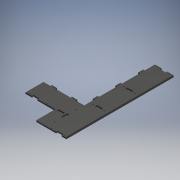
# Autodesk Inventor part: BA10
Saved by Autodesk Inventor 2017 (Build 210142000, 142)
## iProperties
Created: 2019-05-29
Part Number: BA10
Material: Wood (Cherry)
Document SubType Name: Modeling
Designer: Dell
Density: 0.63 g/cm^3
Appearance: Smooth - Black
Mass: 296.487 g
Surface Area: 1614.58 cm^2
Volume: 470.615 cm^3
Author: Dell
Autodesk Inventor part; units mm, degrees
ref_plane "YZ Plane" through (0, 0, 0) normal (1, 0, 0) x (0, 1, 0)
ref_plane "XZ Plane" through (0, 0, 0) normal (0, 1, 0) x (-1, 0, 0)
ref_plane "XY Plane" through (0, 0, 0) normal (0, 0, 1) x (1, 0, 0)
sketch "Sketch1" plane through (0, 0, 0) normal (0, 0, 1) x (1, 0, 0)
  line L0 (0, 0) -> (0, 355.6)
  line L1 (0, 355.6) -> (95.25, 355.6)
  line L2 (95.25, 355.6) -> (95.25, -184.15)
  line L3 (95.25, -184.15) -> (-208.3092, -184.15) construction
  line L4 (-208.3092, -184.15) -> (-208.3092, 0) construction
  line L5 (-208.3092, 0) -> (0, 0)
  line L6 (-208.3092, -184.15) -> (-55.9092, -184.15) construction
  line L7 (-55.9092, -184.15) -> (-55.9092, -88.9)
  line L8 (-55.9092, -88.9) -> (-208.3092, -88.9)
  line L9 (-208.3092, -88.9) -> (-208.3092, -184.15) construction
  line L10 (-208.3092, -88.9) -> (-208.3092, 0)
  line L11 (-55.9092, -184.15) -> (95.25, -184.15)
  line L12 (0, 304.8) -> (-7.62, 304.8)
  line L13 (-7.62, 304.8) -> (-7.62, 279.4)
  line L14 (-7.62, 279.4) -> (0, 279.4)
  line L15 (0, 279.4) -> (0, 304.8)
  line L16 (0, 165.1) -> (-7.62, 165.1)
  line L17 (-7.62, 165.1) -> (-7.62, 190.5)
  line L18 (-7.62, 190.5) -> (0, 190.5)
  line L19 (0, 190.5) -> (0, 165.1)
  line L20 (0, 76.2) -> (-7.62, 76.2)
  line L21 (-7.62, 76.2) -> (-7.62, 50.8)
  line L22 (-7.62, 50.8) -> (0, 50.8)
  line L23 (0, 50.8) -> (0, 76.2)
  line L24 (-6.35, -79.375) -> (0, -79.375)
  line L25 (0, -79.375) -> (0, -104.775)
  line L26 (0, -104.775) -> (-6.35, -104.775)
  line L27 (-6.35, -104.775) -> (-6.35, -79.375)
  line L28 (-7.62, -78.105) -> (1.27, -78.105)
  line L29 (1.27, -78.105) -> (1.27, -106.045)
  line L30 (1.27, -106.045) -> (-7.62, -106.045)
  line L31 (-7.62, -106.045) -> (-7.62, -78.105)
  point P0 (0, 177.8)
  point P1 (0, -92.075)
  point P2 (-6.35, -92.075)
  point P3 (-7.62, -92.075)
  point P4 (-3.175, -79.375)
  point P5 (-3.175, -78.105)
  point P6 (-208.3092, -92.075)
  dimension "d0" = 95.25
  dimension "d1" = 355.6
  dimension "d2" = 303.5592
  dimension "d3" = 184.15
  dimension "d4" = 152.4
  dimension "d5" = 95.25
  dimension "d6" = 7.62
  dimension "d7" = 25.4
  dimension "d8" = 25.4
  dimension "d9" = 25.4
  dimension "d10" = 50.8
  dimension "d11" = 50.8
  dimension "d12" = 6.35
  dimension "d13" = 25.4
  dimension "d14" = 1.27
  dimension "d15" = 1.27
  constraints: 64 end point, 12 parallel, 10 perpendicular, 8 midpoint, 7 horizontal, 4 point on line, 3 vertical alignment, 2 horizontal alignment, 2 vertical, 1 collinear
  measures "d0" distance between parallel lines of L2 L0
  measures "d1" distance of L0.start L0.end
  measures "d2" distance between parallel lines of L4 L2
  measures "d3" distance of L3.end L4.end
  measures "d4" distance of L7.end L8.end
  measures "d5" distance of L6.end L7.end
  measures "d6" distance of L14.end L13.end
  measures "d7" distance of L12.end L13.end
  measures "d8" distance of L16.end L17.end
  measures "d9" distance of L20.end L21.end
  measures "d10" distance between parallel lines of L1 L12
  measures "d11" distance between parallel lines of L5 L22
  measures "d12" distance of L25.end L26.end
  measures "d13" distance of L24.end L25.end
  measures "d14" distance between parallel lines of L28 L24
  measures "d15" distance between parallel lines of L29 L25
extrude "Extrusion1" add sketch "Sketch1" along normal blind 6.35 contours L0 L1 L2 L11 L7 L8 L10 L5 | L22 L21 L20 L0 | L16 L17 L18 L0 | L14 L13 L12 L0
sketch "Sketch3" plane through (0, 355.6, 0) normal (0, 1, 0) x (1, 0, 0)
  line L0 (95.25, 0) -> (95.25, -6.35) projected
  line L1 (95.25, 0) -> (91.5838, -6.35)
  line L2 (91.5838, -6.35) -> (95.25, -6.35)
  line L3 (95.25, -6.35) -> (91.5838, -6.35)
  line L4 (-208.3092, 0) -> (-208.3092, -6.35)
  line L5 (-208.3092, -6.35) -> (-204.6431, -6.35)
  line L6 (-208.3092, 0) -> (-208.3092, -6.35) projected
  line L7 (-204.6431, -6.35) -> (-208.3092, 0)
  line L8 (0, -6.35) -> (-208.3092, -6.35) projected
  line L9 (95.25, -6.35) -> (0, -6.35) projected
  dimension "d23" = 30
  dimension "d24" = 30
  constraints: 12 end point, 2 point on line, 1 collinear, 1 vertical
  measures "d23" angle of L0 L1
  measures "d24" angle of L4 L7
extrude "Extrusion2" cut sketch "Sketch3" against normal through all
sketch "Sketch4" plane through (0, 0, 6.35) normal (0, 0, 1) x (1, 0, 0)
  line L0 (-55.9092, -184.15) -> (91.5838, -184.15) projected
  line L1 (44.45, -184.15) -> (69.85, -184.15)
  line L2 (69.85, -184.15) -> (69.85, -176.53)
  line L3 (69.85, -176.53) -> (44.45, -176.53)
  line L4 (44.45, -176.53) -> (44.45, -184.15)
  line L5 (-7.62, -106.045) -> (-7.62, -78.105) projected
  point P0 (0, 0)
  dimension "d25" = 25.4
  dimension "d26" = 7.62
  dimension "d27" = 52.07
  constraints: 8 end point, 2 parallel, 1 horizontal, 1 perpendicular, 1 point on line
  measures "d25" distance of L3.end L2.end
  measures "d26" distance of L2.end L1.end
  measures "d27" distance between parallel lines of L4 L5
extrude "Extrusion3" cut sketch "Sketch4" against normal through all
sketch "Sketch5" plane through (0, 0, 6.35) normal (0, 0, 1) x (1, 0, 0)
  line L0 (33.0919, 355.6) -> (58.4919, 355.6)
  line L1 (58.4919, 355.6) -> (58.4919, 347.98)
  line L2 (58.4919, 347.98) -> (33.0919, 347.98)
  line L3 (33.0919, 347.98) -> (33.0919, 355.6)
  line L4 (91.5838, 355.6) -> (0, 355.6) projected
  point P0 (0, 0)
  point P1 (45.7919, 355.6)
  dimension "d30" = 7.62
  dimension "d31" = 25.4
  constraints: 8 end point, 2 midpoint, 2 parallel, 1 horizontal, 1 perpendicular
  measures "d30" distance of L2.end L0.start
  measures "d31" distance of L1.end L2.end
extrude "Extrusion4" cut sketch "Sketch5" against normal through all
sketch "Sketch6" plane through (0, 0, 6.35) normal (0, 0, 1) x (1, 0, 0)
  line L0 (33.0919, 31.75) -> (58.4919, 31.75)
  line L1 (58.4919, 31.75) -> (58.4919, 25.4)
  line L2 (58.4919, 25.4) -> (33.0919, 25.4)
  line L3 (33.0919, 25.4) -> (33.0919, 31.75)
  line L4 (-55.9092, -184.15) -> (44.45, -184.15) projected
  line L5 (58.4919, 347.98) -> (33.0919, 347.98) projected
  point P0 (0, 0)
  point P1 (45.7919, 31.75)
  point P2 (45.7919, 347.98)
  dimension "d34" = 25.4
  dimension "d35" = 6.35
  dimension "d36" = 209.55
  constraints: 8 end point, 2 midpoint, 2 parallel, 1 horizontal, 1 perpendicular, 1 vertical alignment
  measures "d34" distance of L1.end L2.end
  measures "d35" distance of L0.end L1.end
  measures "d36" distance between parallel lines of L4 L2
extrude "Extrusion5" cut sketch "Sketch6" against normal through all
sketch "Sketch7" plane through (0, 0, 6.35) normal (0, 0, 1) x (1, 0, 0)
  line L0 (33.0919, 184.15) -> (58.4919, 184.15)
  line L1 (58.4919, 184.15) -> (58.4919, 177.8)
  line L2 (58.4919, 177.8) -> (33.0919, 177.8)
  line L3 (33.0919, 177.8) -> (33.0919, 184.15)
  line L4 (58.4919, 347.98) -> (33.0919, 347.98) projected
  line L5 (33.0919, 355.6) -> (0, 355.6) projected
  point P0 (0, 0)
  point P1 (45.7919, 184.15)
  point P2 (45.7919, 347.98)
  dimension "d39" = 25.4
  dimension "d40" = 6.35
  dimension "d41" = 177.8
  constraints: 8 end point, 2 midpoint, 2 parallel, 1 horizontal, 1 perpendicular, 1 vertical alignment
  measures "d39" distance of L1.end L2.end
  measures "d40" distance of L0.end L1.end
  measures "d41" distance between parallel lines of L5 L2
extrude "Extrusion6" cut sketch "Sketch7" against normal through all
sketch "Sketch8" plane through (0, 0, 6.35) normal (0, 0, 1) x (1, 0, 0)
  line L0 (-170.2092, 0) -> (-144.8092, 0)
  line L1 (-144.8092, 0) -> (-144.8092, 7.62)
  line L2 (-144.8092, 7.62) -> (-170.2092, 7.62)
  line L3 (-170.2092, 7.62) -> (-170.2092, 0)
  line L4 (-68.6092, 0) -> (-43.2092, 0)
  line L5 (-43.2092, 0) -> (-43.2092, 7.62)
  line L6 (-43.2092, 7.62) -> (-68.6092, 7.62)
  line L7 (-68.6092, 7.62) -> (-68.6092, 0)
  line L8 (-157.5092, 7.62) -> (-55.9092, 7.62) construction
  line L9 (0, 0) -> (-208.3092, 0) projected
  dimension "d44" = 25.4
  dimension "d45" = 7.62
  dimension "d46" = 25.4
  dimension "d47" = 7.62
  dimension "d48" = 101.6
  dimension "d51" = 38.1
  constraints: 18 end point, 4 parallel, 2 horizontal, 2 midpoint, 2 perpendicular, 2 point on line
  measures "d44" distance of L2.end L1.end
  measures "d45" distance of L1.end L0.end
  measures "d46" distance of L6.end L5.end
  measures "d47" distance of L5.end L4.end
  measures "d48" distance of L8.start L8.end
  measures "d51" horizontal distance of L2.end L9.end
extrude "Extrusion7" add sketch "Sketch8" against normal blind 6.35
sketch "Sketch9" plane through (0, 0, 6.35) normal (0, 0, 1) x (1, 0, 0)
  line L0 (33.0919, 28.575) -> (0, 28.575) construction
  line L1 (0, 50.8) -> (0, 0) construction
  line L2 (58.4919, 28.575) -> (91.5838, 28.575) construction
  line L3 (91.5838, -184.15) -> (91.5838, 355.6) construction
  circle A0 centre (16.546, 28.575) radius 2.25
  circle A1 centre (75.0379, 28.575) radius 2.25
  line L4 (33.0919, 25.4) -> (33.0919, 31.75) projected
  line L5 (58.4919, 31.75) -> (58.4919, 25.4) projected
  circle A2 centre (16.546, 180.975) radius 2.25
  circle A3 centre (75.0379, 180.975) radius 2.25
  line L6 (58.4919, 184.15) -> (58.4919, 177.8) projected
  circle A4 centre (16.546, 351.79) radius 2.25
  circle A5 centre (75.0379, 351.79) radius 2.25
  line L7 (33.0919, 347.98) -> (33.0919, 355.6) projected
  circle A6 centre (-3.175, -39.0525) radius 2.25
  circle A7 centre (-3.175, -145.0975) radius 2.25
  line L8 (1.27, -106.045) -> (-7.62, -106.045) construction
  line L9 (-7.62, -78.105) -> (1.27, -78.105) construction
  line L10 (-3.175, -78.105) -> (-3.175, 0) construction
  line L11 (-3.175, -106.045) -> (-3.175, -184.15) construction
  line L12 (-55.9092, -184.15) -> (44.45, -184.15) construction
  line L13 (0, 0) -> (-43.2092, 0) projected
  circle A8 centre (-157.5092, 3.81) radius 2.25
  circle A9 centre (-55.9092, 3.81) radius 2.25
  circle A10 centre (-3.81, 63.5) radius 2.25
  circle A11 centre (-3.81, 177.8) radius 2.25
  circle A12 centre (-3.81, 292.1) radius 2.25
  line L14 (-144.8092, 7.62) -> (-170.2092, 7.62) projected
  line L15 (-43.2092, 7.62) -> (-68.6092, 7.62) projected
  line L16 (-7.62, 304.8) -> (-7.62, 279.4) projected
  line L17 (-7.62, 190.5) -> (-7.62, 165.1) projected
  line L18 (-7.62, 76.2) -> (-7.62, 50.8) projected
  line L19 (-68.6092, 7.62) -> (-68.6092, 0) projected
  line L20 (-7.62, 50.8) -> (0, 50.8) projected
  circle A13 centre (16.546, -180.34) radius 2.25
  circle A14 centre (80.7169, -180.34) radius 2.25
  line L21 (69.85, -176.53) -> (69.85, -184.15) projected
  line L22 (69.85, -180.34) -> (91.5838, -180.34) construction
  point P0 (58.4919, 180.975)
  point P1 (33.0919, 351.79)
  point P2 (-3.175, -145.0975)
  point P3 (-157.5092, 7.62)
  point P4 (-55.9092, 7.62)
  point P5 (-7.62, 292.1)
  point P6 (-7.62, 177.8)
  point P7 (-7.62, 63.5)
  point P8 (-68.6092, 3.81)
  point P9 (-3.81, 50.8)
  dimension "d52" = 4.5
  dimension "d53" = 4.5
  dimension "d54" = 4.5
  dimension "d55" = 4.5
  dimension "d56" = 4.5
  dimension "d57" = 4.5
  dimension "d58" = 4.5
  dimension "d59" = 4.5
  dimension "d60" = 4.5
  dimension "d61" = 4.5
  dimension "d62" = 4.5
  dimension "d63" = 4.5
  dimension "d64" = 4.5
  dimension "d65" = 4.5
  dimension "d66" = 4.5
  constraints: 19 midpoint, 15 centre point, 12 vertical alignment, 11 horizontal alignment, 10 end point, 7 point on line, 3 coincident, 2 vertical, 1 horizontal, 1 perpendicular
  measures "d52" diameter of A0
  measures "d53" diameter of A1
  measures "d54" diameter of A2
  measures "d55" diameter of A3
  measures "d56" diameter of A4
  measures "d57" diameter of A5
  measures "d58" diameter of A6
  measures "d59" diameter of A7
  measures "d60" diameter of A8
  measures "d61" diameter of A9
  measures "d62" diameter of A10
  measures "d63" diameter of A11
  measures "d64" diameter of A12
  measures "d65" diameter of A13
  measures "d66" diameter of A14
extrude "Extrusion8" cut sketch "Sketch9" against normal through all
sketch "Sketch10" plane through (0, 0, 6.35) normal (0, 0, 1) x (1, 0, 0)
  line L0 (-171.4646, -82.55) -> (-146.0646, -82.55)
  line L1 (-146.0646, -82.55) -> (-146.0646, -88.9)
  line L2 (-146.0646, -88.9) -> (-171.4646, -88.9)
  line L3 (-171.4646, -88.9) -> (-171.4646, -82.55)
  line L4 (-19.0646, -82.55) -> (-44.4646, -82.55)
  line L5 (-44.4646, -82.55) -> (-44.4646, -88.9)
  line L6 (-44.4646, -88.9) -> (-19.0646, -88.9)
  line L7 (-19.0646, -88.9) -> (-19.0646, -82.55)
  line L8 (-55.9092, -184.15) -> (44.45, -184.15) projected
  line L9 (-204.6431, -88.9) -> (-55.9092, -88.9) projected
  line L10 (58.4919, 25.4) -> (33.0919, 25.4) projected
  line L11 (-55.9092, -88.9) -> (-7.62, -88.9) construction
  line L12 (-7.62, -78.105) -> (-7.62, -106.045) projected
  point P0 (0, 0)
  point P1 (45.7919, 25.4)
  point P2 (-31.7646, -88.9)
  dimension "d70" = 6.35
  dimension "d71" = 25.4
  dimension "d72" = 25.4
  dimension "d73" = 101.6
  constraints: 18 end point, 4 parallel, 4 point on line, 3 horizontal, 3 midpoint, 2 perpendicular
  measures "d70" distance of L2.end L0.start
  measures "d71" distance of L0.start L0.end
  measures "d72" distance of L4.start L4.end
  measures "d73" distance of L4.end L0.end
extrude "Extrusion9" cut sketch "Sketch10" against normal through all
sketch "Sketch11" plane through (0, 0, 6.35) normal (0, 0, 1) x (1, 0, 0)
  circle A0 centre (-100.9869, -85.725) radius 2.25
  circle A1 centre (-188.0538, -85.725) radius 2.25
  line L0 (-204.6431, -88.9) -> (-171.4646, -88.9) projected
  line L1 (-146.0646, -88.9) -> (-55.9092, -88.9) projected
  line L2 (-171.4646, -88.9) -> (-171.4646, -82.55) projected
  point P0 (0, 0)
  point P1 (-188.0538, -88.9)
  point P2 (-100.9869, -88.9)
  point P3 (-171.4646, -85.725)
  point P4 (-171.4646, -85.725)
  dimension "d76" = 4.5
  dimension "d77" = 4.5
  constraints: 4 midpoint, 2 centre point, 2 horizontal alignment, 2 vertical alignment
  measures "d76" diameter of A0
  measures "d77" diameter of A1
extrude "Extrusion10" cut sketch "Sketch11" against normal through all
sketch "Sketch12" plane through (0, 0, 6.35) normal (0, 0, 1) x (1, 0, 0)
  line L0 (33.0919, 355.6) -> (0, 355.6) projected
  line L1 (31.8219, 355.6) -> (59.7619, 355.6)
  line L2 (59.7619, 355.6) -> (59.7619, 347.98)
  line L3 (59.7619, 347.98) -> (31.8219, 347.98)
  line L4 (31.8219, 347.98) -> (31.8219, 355.6)
  line L5 (31.8219, 185.42) -> (59.7619, 185.42)
  line L6 (59.7619, 185.42) -> (59.7619, 176.53)
  line L7 (59.7619, 176.53) -> (31.8219, 176.53)
  line L8 (31.8219, 176.53) -> (31.8219, 185.42)
  line L9 (31.8219, 33.02) -> (59.7619, 33.02)
  line L10 (59.7619, 33.02) -> (59.7619, 24.13)
  line L11 (59.7619, 24.13) -> (31.8219, 24.13)
  line L12 (31.8219, 24.13) -> (31.8219, 33.02)
  line L13 (-204.6431, -88.9) -> (-171.4646, -88.9) projected
  line L14 (-172.7346, -88.9) -> (-144.7946, -88.9)
  line L15 (-144.7946, -88.9) -> (-144.7946, -81.28)
  line L16 (-144.7946, -81.28) -> (-172.7346, -81.28)
  line L17 (-172.7346, -81.28) -> (-172.7346, -88.9)
  line L18 (-45.7346, -81.28) -> (-17.7946, -81.28)
  line L19 (-17.7946, -81.28) -> (-17.7946, -90.17)
  line L20 (-17.7946, -90.17) -> (-45.7346, -90.17)
  line L21 (-45.7346, -90.17) -> (-45.7346, -81.28)
  line L22 (-55.9092, -184.15) -> (44.45, -184.15) projected
  line L23 (43.18, -184.15) -> (71.12, -184.15)
  line L24 (71.12, -184.15) -> (71.12, -176.53)
  line L25 (71.12, -176.53) -> (43.18, -176.53)
  line L26 (43.18, -176.53) -> (43.18, -184.15)
  line L27 (-171.4646, -82.55) -> (-146.0646, -82.55) projected
  line L28 (-171.4646, -88.9) -> (-171.4646, -82.55) projected
  line L29 (-44.4646, -88.9) -> (-44.4646, -82.55) projected
  line L30 (33.0919, 25.4) -> (33.0919, 31.75) projected
  line L31 (58.4919, 31.75) -> (33.0919, 31.75) projected
  line L32 (33.0919, 177.8) -> (33.0919, 184.15) projected
  line L33 (33.0919, 184.15) -> (58.4919, 184.15) projected
  line L34 (58.4919, 347.98) -> (33.0919, 347.98) projected
  line L35 (44.45, -176.53) -> (69.85, -176.53) projected
  line L36 (44.45, -184.15) -> (44.45, -176.53) projected
  line L37 (-19.0646, -88.9) -> (-44.4646, -88.9) projected
  point P0 (0, 0)
  point P1 (-158.7646, -82.55)
  point P2 (-158.7646, -82.55)
  point P3 (-158.7646, -81.28)
  point P4 (45.7919, 347.98)
  point P5 (45.7919, 184.15)
  point P6 (45.7919, 185.42)
  point P7 (33.0919, 180.975)
  point P8 (31.8219, 180.975)
  point P9 (33.0919, 28.575)
  point P10 (31.8219, 28.575)
  point P11 (45.7919, 31.75)
  point P12 (45.7919, 33.02)
  point P13 (57.15, -176.53)
  point P14 (-31.7646, -88.9)
  point P15 (-31.7646, -90.17)
  point P16 (-44.4646, -85.725)
  point P17 (-45.7346, -85.725)
  dimension "d80" = 1.27
  dimension "d81" = 1.27
  dimension "d82" = 1.27
  dimension "d83" = 1.27
  dimension "d84" = 1.27
  dimension "d85" = 1.27
  dimension "d86" = 1.27
  dimension "d87" = 1.27
  constraints: 48 end point, 19 midpoint, 12 parallel, 6 horizontal, 6 perpendicular, 6 point on line, 4 vertical alignment, 3 horizontal alignment
  measures "d80" distance from line of L27 L15.end
  measures "d81" distance between parallel lines of L17 L28
  measures "d82" distance between parallel lines of L21 L29
  measures "d83" distance between parallel lines of L12 L30
  measures "d84" distance from line of L9.end L31
  measures "d85" distance between parallel lines of L8 L32
  measures "d86" distance between parallel lines of L33 L5
  measures "d87" distance between parallel lines of L26 L36
extrude "Extrusion11" cut sketch "Sketch12" against normal through all
sketch "Sketch13" plane through (0, 0, 6.35) normal (0, 0, 1) x (1, 0, 0)
  line L0 (71.12, -176.53) -> (71.12, -184.15) construction
  line L1 (71.12, -184.15) -> (91.5838, -184.15) construction
  line L2 (91.5838, -184.15) -> (91.5838, 355.6) construction
  line L3 (91.5838, 355.6) -> (59.7619, 355.6) construction
  line L4 (59.7619, 355.6) -> (59.7619, 347.98) construction
  line L5 (59.7619, 347.98) -> (31.8219, 347.98) construction
  line L6 (31.8219, 347.98) -> (31.8219, 355.6) construction
  line L7 (31.8219, 355.6) -> (0, 355.6) construction
  line L8 (0, 355.6) -> (0, 304.8) construction
  line L9 (0, 304.8) -> (-7.62, 304.8) construction
  line L10 (-7.62, 304.8) -> (-7.62, 279.4) construction
  line L11 (-7.62, 279.4) -> (0, 279.4) construction
  line L12 (0, 279.4) -> (0, 190.5) construction
  line L13 (0, 190.5) -> (-7.62, 190.5) construction
  line L14 (-7.62, 190.5) -> (-7.62, 165.1) construction
  line L15 (-7.62, 165.1) -> (0, 165.1) construction
  line L16 (0, 165.1) -> (0, 76.2) construction
  line L17 (0, 76.2) -> (-7.62, 76.2) construction
  line L18 (-7.62, 76.2) -> (-7.62, 50.8) construction
  line L19 (-7.62, 50.8) -> (0, 50.8) construction
  line L20 (0, 50.8) -> (0, 0) construction
  line L21 (0, 0) -> (-43.2092, 0) construction
  line L22 (-43.2092, 0) -> (-43.2092, 7.62) construction
  line L23 (-43.2092, 7.62) -> (-68.6092, 7.62) construction
  line L24 (-68.6092, 7.62) -> (-68.6092, 0) construction
  line L25 (-68.6092, 0) -> (-144.8092, 0) construction
  line L26 (-144.8092, 0) -> (-144.8092, 7.62) construction
  line L27 (-144.8092, 7.62) -> (-170.2092, 7.62) construction
  line L28 (-170.2092, 7.62) -> (-170.2092, 0) construction
  line L29 (-170.2092, 0) -> (-204.6431, 0) construction
  line L30 (-204.6431, 0) -> (-204.6431, -88.9) construction
  line L31 (-204.6431, -88.9) -> (-172.7346, -88.9) construction
  line L32 (-172.7346, -88.9) -> (-172.7346, -81.28) construction
  line L33 (-172.7346, -81.28) -> (-144.7946, -81.28) construction
  line L34 (-144.7946, -81.28) -> (-144.7946, -88.9) construction
  line L35 (-144.7946, -88.9) -> (-55.9092, -88.9) construction
  line L36 (-55.9092, -88.9) -> (-55.9092, -184.15) construction
  line L37 (-55.9092, -184.15) -> (43.18, -184.15) construction
  line L38 (43.18, -184.15) -> (43.18, -176.53) construction
  line L39 (43.18, -176.53) -> (71.12, -176.53) construction
  line L40 (31.8219, 24.13) -> (31.8219, 33.02) construction
  line L41 (31.8219, 33.02) -> (59.7619, 33.02) construction
  line L42 (59.7619, 33.02) -> (59.7619, 24.13) construction
  line L43 (59.7619, 24.13) -> (31.8219, 24.13) construction
  line L44 (31.8219, 176.53) -> (31.8219, 185.42) construction
  line L45 (31.8219, 185.42) -> (59.7619, 185.42) construction
  line L46 (59.7619, 185.42) -> (59.7619, 176.53) construction
  line L47 (59.7619, 176.53) -> (31.8219, 176.53) construction
  line L48 (-45.7346, -90.17) -> (-45.7346, -81.28) construction
  line L49 (-45.7346, -81.28) -> (-17.7946, -81.28) construction
  line L50 (-17.7946, -81.28) -> (-17.7946, -90.17) construction
  line L51 (-17.7946, -90.17) -> (-45.7346, -90.17) construction
  circle A0 centre (-100.9869, -85.725) radius 2.25 construction
  circle A1 centre (-188.0538, -85.725) radius 2.25 construction
  circle A2 centre (16.546, -180.34) radius 2.25 construction
  circle A3 centre (-3.81, 177.8) radius 2.25 construction
  circle A4 centre (-55.9092, 3.81) radius 2.25 construction
  circle A5 centre (-3.175, -145.0975) radius 2.25 construction
  circle A6 centre (75.0379, 351.79) radius 2.25 construction
  circle A7 centre (75.0379, 180.975) radius 2.25 construction
  circle A8 centre (75.0379, 28.575) radius 2.25 construction
  circle A9 centre (16.546, 28.575) radius 2.25 construction
  circle A10 centre (16.546, 180.975) radius 2.25 construction
  circle A11 centre (16.546, 351.79) radius 2.25 construction
  circle A12 centre (-3.175, -39.0525) radius 2.25 construction
  circle A13 centre (-157.5092, 3.81) radius 2.25 construction
  circle A14 centre (-3.81, 63.5) radius 2.25 construction
  circle A15 centre (-3.81, 292.1) radius 2.25 construction
  circle A16 centre (80.7169, -180.34) radius 2.25 construction
  line L52 (1.27, -78.105) -> (1.27, -106.045) construction
  line L53 (1.27, -106.045) -> (-7.62, -106.045) construction
  line L54 (-7.62, -106.045) -> (-7.62, -78.105) construction
  line L55 (-7.62, -78.105) -> (1.27, -78.105) construction
  line L56 (-2.2451, 192.7451) -> (-2.2451, 277.1549) construction
  line L57 (-2.2451, 277.1549) -> (-9.8651, 277.1549) construction
  line L58 (-9.8651, 277.1549) -> (-9.8651, 307.0451) construction
  line L59 (-9.8651, 307.0451) -> (-2.2451, 307.0451) construction
  line L60 (-2.2451, 307.0451) -> (-2.2451, 357.8451) construction
  line L61 (-2.2451, 357.8451) -> (34.067, 357.8451) construction
  line L62 (34.067, 357.8451) -> (34.067, 350.2251) construction
  line L63 (34.067, 350.2251) -> (57.5168, 350.2251) construction
  line L64 (57.5168, 350.2251) -> (57.5168, 357.8451) construction
  line L65 (57.5168, 357.8451) -> (93.8289, 357.8451) construction
  line L66 (93.8289, 357.8451) -> (93.8289, -186.3951) construction
  line L67 (93.8289, -186.3951) -> (68.8749, -186.3951) construction
  line L68 (68.8749, -186.3951) -> (68.8749, -178.7751) construction
  line L69 (68.8749, -178.7751) -> (45.4251, -178.7751) construction
  line L70 (45.4251, -178.7751) -> (45.4251, -186.3951) construction
  line L71 (45.4251, -186.3951) -> (-58.1543, -186.3951) construction
  line L72 (-58.1543, -186.3951) -> (-58.1543, -91.1451) construction
  line L73 (-58.1543, -91.1451) -> (-147.0397, -91.1451) construction
  line L74 (-147.0397, -91.1451) -> (-147.0397, -83.5251) construction
  line L75 (-147.0397, -83.5251) -> (-170.4895, -83.5251) construction
  line L76 (-170.4895, -83.5251) -> (-170.4895, -91.1451) construction
  line L77 (-170.4895, -91.1451) -> (-206.8881, -91.1451) construction
  line L78 (-206.8881, -91.1451) -> (-206.8881, 2.2451) construction
  line L79 (-206.8881, 2.2451) -> (-172.4543, 2.2451) construction
  line L80 (-172.4543, 2.2451) -> (-172.4543, 9.8651) construction
  line L81 (-172.4543, 9.8651) -> (-142.5642, 9.8651) construction
  line L82 (-142.5642, 9.8651) -> (-142.5642, 2.2451) construction
  line L83 (-142.5642, 2.2451) -> (-70.8543, 2.2451) construction
  line L84 (-70.8543, 2.2451) -> (-70.8543, 9.8651) construction
  line L85 (-70.8543, 9.8651) -> (-40.9642, 9.8651) construction
  line L86 (-40.9642, 9.8651) -> (-40.9642, 2.2451) construction
  line L87 (-40.9642, 2.2451) -> (-2.2451, 2.2451) construction
  line L88 (-2.2451, 2.2451) -> (-2.2451, 48.5549) construction
  line L89 (-2.2451, 48.5549) -> (-9.8651, 48.5549) construction
  line L90 (-9.8651, 48.5549) -> (-9.8651, 78.4451) construction
  line L91 (-9.8651, 78.4451) -> (-2.2451, 78.4451) construction
  line L92 (-2.2451, 78.4451) -> (-2.2451, 162.8549) construction
  line L93 (-2.2451, 162.8549) -> (-9.8651, 162.8549) construction
  line L94 (-9.8651, 162.8549) -> (-9.8651, 192.7451) construction
  line L95 (-9.8651, 192.7451) -> (-2.2451, 192.7451) construction
  line L96 (0, 0) -> (-43.2092, 0) projected
  circle A17 centre (-2.2451, 2.2451) radius 3.175
  circle A18 centre (-40.9642, 2.2451) radius 3.175
  circle A19 centre (-70.8543, 2.2451) radius 3.175
  circle A20 centre (-172.4543, 2.2451) radius 3.175
  circle A21 centre (-142.5642, 2.2451) radius 3.175
  line L97 (-172.7346, -81.28) -> (-144.7946, -81.28) projected
  circle A22 centre (-170.4895, -83.5251) radius 3.175
  circle A23 centre (-147.0397, -83.5251) radius 3.175
  line L98 (43.18, -184.15) -> (43.18, -176.53) projected
  circle A24 centre (45.4251, -178.7751) radius 3.175
  circle A25 centre (68.8749, -178.7751) radius 3.175
  line L99 (0, 50.8) -> (0, 0) projected
  circle A26 centre (-2.2451, 48.5549) radius 3.175
  line L100 (0, 165.1) -> (0, 76.2) projected
  circle A27 centre (-2.2451, 78.4451) radius 3.175
  circle A28 centre (-2.2451, 162.8549) radius 3.175
  circle A29 centre (-2.2451, 192.7451) radius 3.175
  line L101 (0, 279.4) -> (0, 190.5) projected
  circle A30 centre (-2.2451, 277.1549) radius 3.175
  circle A31 centre (-2.2451, 307.0451) radius 3.175
  circle A32 centre (34.067, 350.2251) radius 3.175
  circle A33 centre (57.5168, 350.2251) radius 3.175
  line L102 (-20.0397, -83.5251) -> (-43.4895, -83.5251) construction
  line L103 (-43.4895, -83.5251) -> (-43.4895, -87.9249) construction
  line L104 (-43.4895, -87.9249) -> (-20.0397, -87.9249) construction
  line L105 (-20.0397, -87.9249) -> (-20.0397, -83.5251) construction
  line L106 (-5.3749, -80.3501) -> (-5.3749, -103.7999) construction
  line L107 (-5.3749, -103.7999) -> (-0.9751, -103.7999) construction
  line L108 (-0.9751, -103.7999) -> (-0.9751, -80.3501) construction
  line L109 (-0.9751, -80.3501) -> (-5.3749, -80.3501) construction
  line L110 (34.067, 26.3751) -> (34.067, 30.7749) construction
  line L111 (34.067, 30.7749) -> (57.5168, 30.7749) construction
  line L112 (57.5168, 30.7749) -> (57.5168, 26.3751) construction
  line L113 (57.5168, 26.3751) -> (34.067, 26.3751) construction
  line L114 (34.067, 178.7751) -> (34.067, 183.1749) construction
  line L115 (34.067, 183.1749) -> (57.5168, 183.1749) construction
  line L116 (57.5168, 183.1749) -> (57.5168, 178.7751) construction
  line L117 (57.5168, 178.7751) -> (34.067, 178.7751) construction
  circle A34 centre (57.5168, 183.1749) radius 3.175
  circle A35 centre (57.5168, 178.7751) radius 3.175
  circle A36 centre (34.067, 183.1749) radius 3.175
  circle A37 centre (34.067, 178.7751) radius 3.175
  line L118 (59.7619, 33.02) -> (31.8219, 33.02) projected
  circle A38 centre (34.067, 30.7749) radius 3.175
  circle A39 centre (34.067, 26.3751) radius 3.175
  line L119 (59.7619, 24.13) -> (31.8219, 24.13) projected
  circle A40 centre (57.5168, 26.3751) radius 3.175
  circle A41 centre (57.5168, 30.7749) radius 3.175
  line L120 (-45.7346, -81.28) -> (-17.7946, -81.28) projected
  circle A42 centre (-20.0397, -83.5251) radius 3.175
  circle A43 centre (-20.0397, -87.9249) radius 3.175
  circle A44 centre (-43.4895, -87.9249) radius 3.175
  circle A45 centre (-43.4895, -83.5251) radius 3.175
  line L121 (-7.62, -78.105) -> (1.27, -78.105) projected
  circle A46 centre (-5.3749, -80.3501) radius 3.175
  circle A47 centre (-0.9751, -80.3501) radius 3.175
  line L122 (1.27, -78.105) -> (1.27, -106.045) projected
  circle A48 centre (-0.9751, -103.7999) radius 3.175
  circle A49 centre (-5.3749, -103.7999) radius 3.175
  dimension "d90" = 6.35
  dimension "d91" = 6.35
  dimension "d92" = 6.35
  dimension "d93" = 6.35
  dimension "d94" = 6.35
  constraints: 112 end point, 33 coincident, 150 other
extrude "Extrusion12" cut sketch "Sketch13" against normal through all contours A17 L96 | L99 A17 | L96 A17 L99 | A18 L96 | L96 A18 | A19 | A20 | A21 | A22 L97 | L97 A22 | A23 L97 | L97 A23 | A24 L98 | L98 A24 | A25 | A26 L99 | L99 A26 | A28 L100 | L100 A28 | A27 L100 | L100 A27 | L101 A29 | A29 L101 | A30 L101 | L101 A30 | A31 | A32 | A33 | A34 A35 | A35 A34 | A34 A35 | A36 A37 | A37 A36 | A36 A37 | A41 A40 L118 | L118 A41 | A38 A39 L118 | L118 A38 | A41 A40 L119 | A40 A41 | L119 A40 | A39 A38 | A38 A39 L119 | A39 L119 | A45 L120 | L120 A45 A44 | A45 A44 | A44 A45 | A42 L120 | L120 A42 A43 | A43 A42 | A42 A43 | A46 A47 L121 | L121 A47 A46 | A47 A46 L121 | L121 A46 A47 | A47 L121 A46 | A46 L121 L122 A47 | A47 L122 | A48 L122 | L122 A48 A49 | A49 A48 | A48 A49
sketch "Sketch14" plane through (-55.9092, -184.15, 0) normal (0, -1, 0) x (1, 0, 0)
  line L0 (151.1592, 0) -> (147.4931, 6.35) projected
  line L1 (147.4931, 6.35) -> (146.7598, 6.35)
  line L2 (147.4931, 6.35) -> (115.6711, 6.35) projected
  line L3 (146.7598, 6.35) -> (150.426, 0)
  line L4 (127.0292, 0) -> (151.1592, 0) projected
  line L5 (150.426, 0) -> (151.1592, 0)
  line L6 (-148.7338, 6.35) -> (-152.4, 0) projected
  line L7 (-148.7338, 6.35) -> (-148.0006, 6.35)
  line L8 (-118.7901, 6.35) -> (-148.7338, 6.35) projected
  line L9 (-148.0006, 6.35) -> (-151.6668, 0)
  line L10 (-118.7901, 0) -> (-152.4, 0) projected
  line L11 (-152.4, 0) -> (-151.6668, 0)
  point P0 (55.9092, 0)
  dimension "d97" = 0.635
  dimension "d98" = 0.635
  constraints: 12 end point, 4 point on line, 2 collinear, 2 parallel
  measures "d97" distance between parallel lines of L3 L0
  measures "d98" distance between parallel lines of L6 L9
extrude "Extrusion13" cut sketch "Sketch14" against normal through all
equation "\"d6\" = Panel_Thickness + Fit_Tolerance"
equation "\"d12\" = Panel_Thickness"
equation "\"d14\" = Fit_Tolerance"
equation "\"d15\" = Fit_Tolerance"
equation "\"d16\" = Panel_Thickness"
equation "\"d26\" = Panel_Thickness + Fit_Tolerance"
equation "\"d30\" = Panel_Thickness + Fit_Tolerance"
equation "\"d35\" = Panel_Thickness"
equation "\"d40\" = Panel_Thickness"
equation "\"d45\" = Panel_Thickness + Fit_Tolerance"
equation "\"d47\" = Panel_Thickness + Fit_Tolerance"
equation "\"d49\" = Panel_Thickness"
equation "\"d67\" = Panel_Thickness"
equation "\"d70\" = Panel_Thickness"
equation "\"d74\" = Panel_Thickness"
equation "\"d78\" = Panel_Thickness"
equation "\"d80\" = Fit_Tolerance"
equation "\"d81\" = Fit_Tolerance"
equation "\"d82\" = Fit_Tolerance"
equation "\"d83\" = Fit_Tolerance"
equation "\"d84\" = Fit_Tolerance"
equation "\"d85\" = Fit_Tolerance"
equation "\"d86\" = Fit_Tolerance"
equation "\"d87\" = Fit_Tolerance"
equation "\"d88\" = Panel_Thickness"
equation "\"d90\" = Tool_Dia"
equation "\"d91\" = Tool_Dia"
equation "\"d92\" = Tool_Dia"
equation "\"d93\" = Tool_Dia"
equation "\"d94\" = Tool_Dia"
equation "\"d95\" = Panel_Thickness"
equation "\"d97\" = 0.5 * Fit_Tolerance"
equation "\"d98\" = 0.5 * Fit_Tolerance"
equation "\"d99\" = Panel_Thickness"
equation "\"Panel_Thickness\" = 6.35"
equation "\"Fit_Tolerance\" = 1.27"
equation "\"Tool_Dia\" = 6.35"
body "Solid1"
